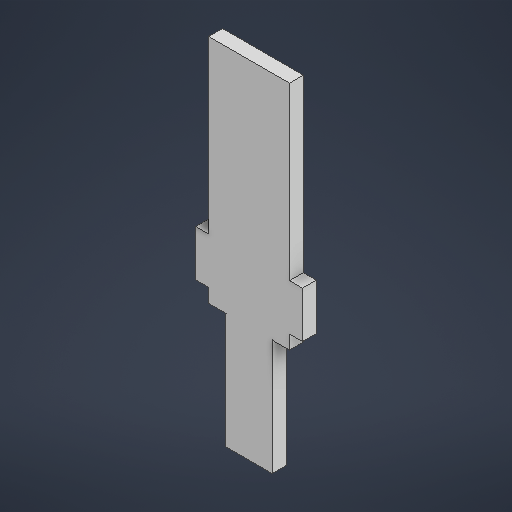
# Autodesk Inventor part: contact_board3
Saved by Autodesk Inventor 2027 (Build 310192000, 192)
## iProperties
Created: 2026-05-11
Part Number: contact_board3
Material: Generic
Document SubType Name: Modeling
Designer: alexy
Density: 1 g/cm^3
Appearance: Default
Author: alexy
Autodesk Inventor part; units mm, degrees
ref_plane "YZ Plane" through (0, 0, 0) normal (1, 0, 0) x (0, 1, 0)
ref_plane "XZ Plane" through (0, 0, 0) normal (0, 1, 0) x (-1, 0, 0)
ref_plane "XY Plane" through (0, 0, 0) normal (0, 0, 1) x (1, 0, 0)
sketch "Sketch1" plane through (0, 0, 0) normal (0, 0, 1) x (1, 0, 0)
  line L0 (0, 0) -> (17.5, 0)
  line L1 (17.5, 0) -> (17.5, 50)
  line L2 (17.5, 50) -> (0, 50)
  line L3 (0, 50) -> (0, 0)
  line L4 (3.75, -25) -> (13.75, -25)
  line L5 (13.75, -25) -> (13.75, 0)
  line L6 (13.75, 0) -> (3.75, 0)
  line L7 (3.75, 0) -> (3.75, -25)
  line L8 (3.75, -25) -> (13.75, 0) construction
  line L9 (13.75, -25) -> (3.75, 0) construction
  line L10 (0, 3) -> (-2.8, 3)
  line L11 (-2.8, 3) -> (-2.8, 13)
  line L12 (-2.8, 13) -> (0, 13)
  line L13 (0, 13) -> (0, 3)
  line L14 (17.5, 3) -> (20.3, 3)
  line L15 (20.3, 3) -> (20.3, 13)
  line L16 (20.3, 13) -> (17.5, 13)
  line L17 (17.5, 13) -> (17.5, 3)
  line L18 (3.75, -25) -> (13.75, -25)
  point P0 (8.75, -12.5)
  point P1 (8.75, 0)
  point P2 (3.75, 0)
  point P3 (17.5, 13)
  point P4 (0, 13)
  dimension "d0" = 17.5
  dimension "d1" = 10
  dimension "d2" = 25
  dimension "d3" = 3
  dimension "d4" = 10
  dimension "d5" = 2.8
  dimension "d6" = 2.8
  dimension "d7" = 50
  constraints: 38 end point, 8 parallel, 5 horizontal, 4 perpendicular, 3 midpoint, 3 point on line, 2 horizontal alignment, 1 vertical alignment
  measures "d0" distance of L0.start L0.end
  measures "d1" distance of L4.start L4.end
  measures "d2" distance of L4.end L5.end
  measures "d3" distance from line of L0.start L10
  measures "d4" distance of L10.end L11.end
  measures "d5" distance of L10.start L10.end
  measures "d6" distance of L14.start L14.end
  measures "d7" distance of L0.end L1.end
extrude "Extrusion1" add sketch "Sketch1" along normal blind 3
body "Solid1"
